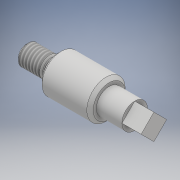
# Autodesk Inventor part: Вал Курганова
Saved by Autodesk Inventor 2017 (Build 210142000, 142)
## iProperties
Part Number: Вал Курганова
Material: Типовые
Document SubType Name: Modeling
Designer: Sasha
Density: 1 g/cm^3
Appearance: По умолчанию
Mass: 45.7168 g
Surface Area: 93.2054 cm^2
Volume: 45.7168 cm^3
Author: Sasha
Autodesk Inventor part; units mm, degrees
ref_plane "YZ Plane" through (0, 0, 0) normal (1, 0, 0) x (0, 1, 0)
ref_plane "XY Plane" through (0, 0, 0) normal (0, 0, 1) x (1, 0, 0)
sketch "Эскиз1" plane through (0, 0, 0) normal (0, 0, 1) x (1, 0, 0)
  line L0 (0, 0) -> (0, 8)
  line L1 (0, 8) -> (18.5, 8)
  line L2 (18.5, 8) -> (20, 6.5)
  line L3 (20, 6.5) -> (25, 6.5)
  line L4 (25, 6.5) -> (25, 15)
  line L5 (25, 15) -> (65, 15)
  line L6 (65, 15) -> (65, 10)
  line L7 (65, 10) -> (85, 10)
  line L8 (85, 10) -> (85, 0)
  line L9 (85, 0) -> (0, 0)
  dimension "d0" = 8
  dimension "d1" = 85
  dimension "d2" = 40
  dimension "d3" = 5
  dimension "d6" = 5
  dimension "d7" = 6.5
  dimension "d8" = 25
  dimension "d9" = 10
  dimension "d10" = 135
  constraints: 20 end point, 6 perpendicular, 1 horizontal, 1 parallel, 1 vertical
  measures "d0" distance of L0.start L0.end
  measures "d1" distance of L8.end L0.start
  measures "d2" distance of L4.end L5.end
  measures "d3" distance of L5.end L6.end
  measures "d6" distance of L2.end L3.end
  measures "d7" distance between parallel lines of L9 L3
  measures "d8" distance between parallel lines of L4 L0
  measures "d9" distance of L7.end L8.end
  measures "d10" angle of L1 L2
revolve "Вращение1" add sketch "Эскиз1" angle 360 about axis through (85, 0, 0) along (-1, 0, 0)
chamfer "Фаска1" distance 2 angle 45 1 edges at (0, -8, 0)
chamfer "Фаска2" distance 2.5 angle 45 2 edges at (25, -15, 0) (65, -15, 0)
fillet "Сопряжение1" radius 1.6 1 edges at (25, -6.5, 0)
fillet "Сопряжение2" radius 1 1 edges at (20, -6.5, 0)
thread "Резьба1" size "M20x2.5" class "6g" standard "ANSI Metric M Profile" full length
sketch "Эскиз2" plane through (85, 0, 0) normal (1, 0, 0) x (0, 0, -1)
  circle A0 centre (0, 0) radius 10 projected
  circle A1 centre (0, 0) radius 12.5 projected
  circle A2 centre (0, 0) radius 15 projected
  line L0 (-8.8388, 8.8388) -> (8.8388, 8.8388)
  line L1 (8.8388, 8.8388) -> (8.8388, -8.8388)
  line L2 (8.8388, -8.8388) -> (-8.8388, -8.8388)
  line L3 (-8.8388, -8.8388) -> (-8.8388, 8.8388)
  point P0 (-7.0711, 7.0711)
  constraints: 8 end point, 3 point on circle, 2 parallel, 2 perpendicular, 1 horizontal
extrude "Выдавливание1" [suppressed]
sketch "Эскиз3" plane through (0, 0, 0) normal (0, 1, 0) x (-1, 0, 0)
  point P0 (0, 0)
ref_plane "РабПлоскость1" through (0, 15, 0) normal (0, 1, 0) x (-1, 0, 0)
sketch "Эскиз4" plane through (0, 15, 0) normal (0, 1, 0) x (-1, 0, 0)
  line L0 (-38.4152, -3.9615) -> (-50.4152, -3.9615)
  line L1 (-50.4152, 4.0385) -> (-38.4152, 4.0385)
  arc A0 (-38.4152, -3.9615) -> (-34.4152, 0.0385) centre (-38.4152, 0.0385) ccw
  arc A1 (-34.4152, 0.0385) -> (-38.4152, 4.0385) centre (-38.4152, 0.0385) ccw
  arc A2 (-50.4152, 4.0385) -> (-54.4152, 0.0385) centre (-50.4152, 0.0385) ccw
  arc A3 (-54.4152, 0.0385) -> (-50.4152, -3.9615) centre (-50.4152, 0.0385) ccw
  point P0 (0, 0)
  point P1 (-34.4152, -3.9615)
  point P2 (-54.4152, 4.0385)
  point P3 (-54.4152, -3.9615)
  dimension "d25" = 20
  dimension "d26" = 8
  dimension "d27" = 4
  constraints: 8 point on circle, 4 centre point, 4 end point, 4 tangent, 3 equal radius, 3 point on line, 2 horizontal, 1 parallel, 13 other
  measures "d25" distance of point (-34.415, -3.962) point (-54.415, -3.962)
  measures "d26" distance of point (-54.415, -3.962) point (-54.415, 4.038)
  measures "d27" radius of A0
extrude "Выдавливание2" cut sketch "Эскиз4" against normal blind 4
sketch "Эскиз5" plane through (85, 0, 0) normal (1, 0, 0) x (0, 0, -1)
  circle A0 centre (0, 0) radius 10 projected
  line L0 (7.0833, 7.0588) -> (-7.0588, 7.0588)
  line L1 (-7.0588, 7.0588) -> (-7.0588, -7.0833)
  line L2 (-7.0588, -7.0833) -> (7.0833, -7.0833)
  line L3 (7.0833, -7.0833) -> (7.0833, 7.0588)
  constraints: 8 end point, 2 parallel, 2 perpendicular, 2 point on circle, 1 horizontal
extrude "Выдавливание3" [suppressed]
sketch "Эскиз6" plane through (85, 0, 0) normal (1, 0, 0) x (0, 0, -1)
  circle A0 centre (0, 0) radius 10 projected
  line L0 (0, 10) -> (-10, 0)
  line L1 (-10, 0) -> (0, -10)
  line L2 (0, -10) -> (10, 0)
  line L3 (10, 0) -> (0, 10)
  constraints: 8 end point, 2 parallel, 2 point on circle, 1 perpendicular
extrude "Выдавливание4" add sketch "Эскиз6" along normal blind 15 contours L2 L1 L0 L3
